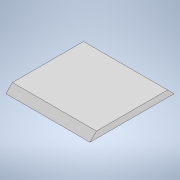
# Autodesk Inventor part: inner_side
Saved by Autodesk Inventor 2021 (Build 250183000, 183)
## iProperties
Created: 2020-06-13
Part Number: inner_side
Material: Generic
Document SubType Name: Modeling
Designer: Yatekii
Density: 1 g/cm^3
Appearance: Default
Author: Yatekii
Autodesk Inventor part; units mm, degrees
ref_plane "YZ Plane" through (0, 0, 0) normal (1, 0, 0) x (0, 1, 0)
ref_plane "XZ Plane" through (0, 0, 0) normal (0, 1, 0) x (-1, 0, 0)
ref_plane "XY Plane" through (0, 0, 0) normal (0, 0, 1) x (1, 0, 0)
sketch "Sketch1" plane through (0, 0, 0) normal (0, 1, 0) x (-1, 0, 0)
  line L0 (-65, -65) -> (65, -65)
  line L1 (65, -65) -> (65, 65)
  line L2 (65, 65) -> (-65, 65)
  line L3 (-65, 65) -> (-65, -65)
  line L4 (-65, -65) -> (65, 65) construction
  line L5 (65, -65) -> (-65, 65) construction
  point P0 (0, 0)
  dimension "d0" = 130
  dimension "d1" = 130
  constraints: 12 end point, 2 midpoint, 2 parallel, 1 horizontal, 1 perpendicular
  measures "d0" distance of L2.end L1.end
  measures "d1" distance of L1.end L0.end
extrude "Extrusion1" add sketch "Sketch1" along normal blind 10
chamfer "Chamfer1" distance 10 angle 45 2 edges at (0, 10, 65) (0, 10, -65)
body "Solid1"
